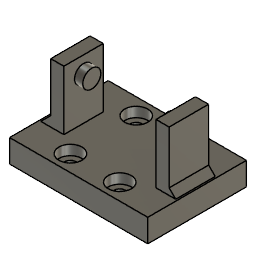
chain mount 1 (Autodesk Fusion 360 design; units mm, degrees)
Autodesk Fusion 360 part; units mm, degrees
sketch "Szkic1" plane through (0, 0, 0) normal (0, 0, 1) x (1, 0, 0)
  line L0 (-23.5, -30) -> (30, -30)
  line L1 (-23.5, 0) -> (-23.5, -30)
  line L2 (30, -30) -> (30, 0)
  line L3 (30, 0) -> (-23.5, 0)
  line L4 (5, -5) -> (7, -5)
  line L5 (18.5, -5) -> (18.5, -30)
  line L6 (18.5, -5) -> (18.5, 0)
  circle A0 centre (5, -25) radius 1.75
  circle A1 centre (5, -5) radius 1.75
  circle A2 centre (-10, -25) radius 1.75
  circle A3 centre (-10, -5) radius 1.75
  circle A4 centre (-10, -25) radius 3.5
  circle A5 centre (5, -25) radius 3.5
  circle A6 centre (5, -5) radius 3.5
  circle A7 centre (-10, -5) radius 3.5
  line L7 (-10, -5) -> (-9, -5)
  line L8 (-9, -5) -> (-2, -5)
  line L9 (-14, -10) -> (-14, -19)
  line L10 (10, -21) -> (10, -9)
  line L11 (10, -9) -> (-14, -9)
  line L12 (-14, -9) -> (-14, -10)
  line L13 (-14, -19) -> (-14, -21)
  line L14 (-14, -21) -> (10, -21)
  dimension "d1" = 13.5
  dimension "d3" = 3.5
  dimension "d4" = 3.5
  dimension "d5" = 3.5
  dimension "d6" = 3.5
  dimension "d7" = 7
  dimension "d8" = 7
  dimension "d9" = 7
  dimension "d10" = 7
  constraint perpendicular L1 L3
  constraint horizontal L4
  constraint coincident L0 L5.end
  constraint perpendicular L0 L5
  constraint coincident L3 L6.end
  constraint perpendicular L3 L6
  constraint concentric A2 A4
  constraint concentric A0 A5
  constraint concentric A1 A6
  constraint concentric A3 A7
  constraint coincident A3.centre A7.centre
  constraint parallel L3 L7
  constraint parallel L4 L8
  constraint vertical L9
  constraint vertical L10
  constraint perpendicular L10 L11
  constraint perpendicular L11 L12
  constraint parallel L9 L13
  constraint perpendicular L10 L14
  measures "d1" distance of L4.start L5.start
  measures "d3" diameter of A0
  measures "d4" diameter of A1
  measures "d5" diameter of A2
  measures "d6" diameter of A3
  measures "d7" diameter of A4
  measures "d8" diameter of A5
  measures "d9" diameter of A6
  measures "d10" diameter of A7
extrude "Wyciągnięcie proste1" add sketch "Szkic1" along normal blind 7 contours L0 L1 L3 L5 L6
extrude "Wyciągnięcie proste2" add sketch "Szkic1" along normal blind 20 contours L9 L10 L11 L12 L13 L14
extrude "Wyciągnięcie proste3" add sketch "Szkic1" along normal blind 4 contours A4 | A5 | A6 | A7
extrude "Wyciągnięcie proste4" add 1 faces at (-6, -13, 20) along direction (0, 0, 1) blind 5
sketch "Szkic2" plane through (10, 0, 0) normal (1, 0, 0) x (0, 1, 0)
  line L0 (-21, 7) -> (-9, 7)
  line L1 (-9, 7) -> (-9, 25)
  line L2 (-9, 25) -> (-21, 25)
  line L3 (-21, 25) -> (-21, 7)
  circle A0 centre (-15, 20) radius 3.25
  dimension "d19" = 6.5
  measures "d19" diameter of A0
extrude "Wyciągnięcie proste5" add sketch "Szkic2" along normal blind 3 contours L0 L1 L2 L3 | A0
extrude "Wyciągnięcie proste6" add 1 faces at (-14, -17, 19) along direction (-1, 0, 0) blind 3
extrude "Wyciągnięcie proste7" cut sketch "Szkic2" against normal blind 24 contours L0 L1 L2 L3 | A0
extrude "Wyciągnięcie proste8" add sketch "Szkic2" against normal blind 22 contours A0
extrude "Wyciągnięcie proste9" add 1 faces at (-12, -14.06, 19.6878) along direction (-1, 0, 0) blind 3
extrude "Wyciągnięcie proste10" cut sketch "Szkic2" against normal blind 21.5 contours A0
extrude "Wyciągnięcie proste11" add sketch "Szkic2" against normal blind 2.5 contours A0
extrude "Wyciągnięcie proste12" cut 1 faces at (-14, -14.919, 10.253) along direction (-1, 0, 0) blind 2
extrude "Wyciągnięcie proste13" cut 1 faces at (10, -14.919, 10.253) along direction (1, 0, 0) blind 2
extrude "Wyciągnięcie proste14" cut 1 faces at (7.5, -14.06, 19.6878) along direction (1, 0, 0) blind 2
extrude "Wyciągnięcie proste15" cut 1 faces at (-11.5, -14.06, 19.6878) along direction (-1, 0, 0) blind 2
extrude "Wyciągnięcie proste16" add 1 faces at (-17, -17, 19) along direction (-1, 0, 0) blind 2
extrude "Wyciągnięcie proste17" add 1 faces at (13, -13, 13) along direction (1, 0, 0) blind 3
extrude "Wyciągnięcie proste18" add 1 faces at (-19, -17, 19) along direction (-1, 0, 0) blind 1
chamfer "Fazowanie1" distance 3 angle 45 1 edges at (-20, -15, 7)
chamfer "Fazowanie2" distance 2 angle 45 1 edges at (16, -15, 7)
sketch "Szkic3" plane through (9.5, 0, 0) normal (-1, 0, 0) x (0, -1, 0)
  circle A0 centre (15, 20) radius 3.25
  circle A1 centre (15, 20) radius 2.75
  dimension "d50" = 5.5
  constraint concentric A0 A1
  measures "d50" diameter of A1
extrude "Wyciągnięcie proste19" cut sketch "Szkic3" against normal blind 2.5
extrude "Wyciągnięcie proste20" cut sketch "Szkic3" along normal blind 25.5
equation "d26 = 2 mm - 24 mm"
